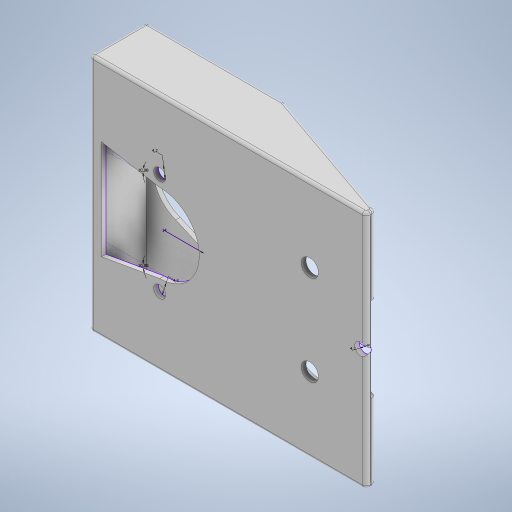
# Autodesk Inventor part: Tower
Saved by Autodesk Inventor 2024 (Build 280153000, 153)
## iProperties
Created: 2025-05-21
Part Number: Tower
Material: Ogólny
Document SubType Name: Modeling
Designer: Victoria
Density: 1 g/cm^3
Appearance: Domyślna
Author: Victoria
Autodesk Inventor part; units mm, degrees
ref_plane "YZ Plane" through (0, 0, 0) normal (1, 0, 0) x (0, 1, 0)
ref_plane "XZ Plane" through (0, 0, 0) normal (0, 1, 0) x (-1, 0, 0)
ref_plane "XY Plane" through (0, 0, 0) normal (0, 0, 1) x (1, 0, 0)
sketch "Szkic1" plane through (0, 0, 0) normal (0, 0, 1) x (1, 0, 0)
  circle A0 centre (0, 16) radius 3
  circle A1 centre (0, -16) radius 3
  line L0 (0, 0) -> (20, 0)
  line L1 (20, 0) -> (20, -42.5)
  line L2 (20, 0) -> (20, 42.5)
  line L3 (20, 0) -> (62.5, 0) construction
  line L4 (20, 42.5) -> (-78, 42.5)
  line L5 (-78, 42.5) -> (-78, -42.5)
  line L6 (-78, -42.5) -> (20, -42.5)
  dimension "d0" = 6
  dimension "d1" = 6
  dimension "d5" = 20
  dimension "d6" = 42.5
  dimension "d7" = 42.5
  dimension "d8" = 90
  dimension "d9" = 98
  dimension "d10" = 85
  dimension "d11" = 90
  constraints: 14 end point, 4 perpendicular, 2 centre point, 2 horizontal, 1 vertical
  measures "d0" diameter of A0
  measures "d1" diameter of A1
  measures "d5" distance of L0.start L0.end
  measures "d6" distance of L0.end L1.end
  measures "d7" distance of L0.end L2.end
  measures "d8" angle of L3 L2
  measures "d9" distance of L2.end L4.end
  measures "d10" distance of L4.end L5.end
  measures "d11" angle of L5 L4
extrude "Wyciągnięcie proste1" add sketch "Szkic1" along normal blind 1.6
sketch "Szkic6" plane through (0, 0, 0) normal (0, 0, -1) x (-1, 0, 0)
  line L0 (-18, 0) -> (53.3, 0)
  circle A0 centre (53.3, -18) radius 2.1
  circle A1 centre (53.3, 18) radius 2.1
  arc A2 (53.3, 14) -> (53.3, -14) centre (53.3, 0) ccw
  line L1 (53.3, -14) -> (74, -17.65)
  line L2 (78, 42.5) -> (78, -42.5) projected
  line L3 (53.3, -14) -> (78.381, -14) construction
  line L4 (53.3, 14) -> (74, 17.65)
  line L5 (53.3, 14) -> (78.381, 14) construction
  line L6 (78, 18.3553) -> (78, -18.3553)
  line L7 (74, -17.65) -> (74, 17.65)
  line L8 (78, 18.3553) -> (78, -18.3553)
  circle A3 centre (-18, 0) radius 2.1
  point P0 (0, 0)
  point P1 (78, 40.5)
  point P2 (78, -40.5)
  point P3 (74, 17.65)
  dimension "d50" = 4.2
  dimension "d52" = 4.2
  dimension "d53" = 14
  dimension "d54" = 10
  dimension "d55" = 10
  dimension "d103" = 4.2
  constraints: 16 end point, 4 centre point, 3 horizontal, 2 coincident, 2 point on circle, 2 point on line, 1 collinear, 1 parallel
  measures "d50" diameter of A0
  measures "d52" diameter of A1
  measures "d53" radius of A2
  measures "d54" angle of L1 L3
  measures "d55" angle of L5 L4
  measures "d103" diameter of A3
extrude "Wyciągnięcie proste6" cut sketch "Szkic6" against normal blind 8
sketch "Szkic15" plane through (0, 0, 0) normal (0, 0, -1) x (-1, 0, 0)
  line L0 (78, -42.5) -> (-20, -42.5) projected
  line L1 (78, -42.5) -> (78, 42.5)
  line L2 (78, 42.5) -> (-20, 42.5)
  line L3 (-20, 42.5) -> (-20, 41)
  line L4 (-20, 41) -> (76.5, 41)
  line L5 (76.5, 41) -> (76.5, -41)
  line L6 (76.5, -41) -> (-20, -41)
  line L7 (-20, -41) -> (-20, -42.5)
  line L8 (-20, -41) -> (-20, -42.5)
  line L9 (-20, -42.5) -> (78, -42.5)
  point P0 (0, 0)
  dimension "d104" = 1.5
  dimension "d105" = 96.5
  dimension "d106" = 82
  constraints: 18 end point, 5 perpendicular, 2 point on line, 1 collinear, 1 parallel
  measures "d104" distance of L2.end L3.end
  measures "d105" distance of L3.end L4.end
  measures "d106" distance of L4.end L5.end
extrude "Wyciągnięcie proste15" add sketch "Szkic15" along normal blind 16.8
sketch "Szkic16" plane through (0, 0, -16.8) normal (0, 0, -1) x (-1, 0, 0)
  line L0 (78, 42.5) -> (-20, 42.5) projected
  line L1 (-20, -42.5) -> (78, -42.5) projected
  line L2 (78, 42.5) -> (-20, 42.5)
  line L3 (-20, 42.5) -> (-20, -42.5)
  line L4 (-20, -42.5) -> (78, -42.5)
  line L5 (78, -42.5) -> (78, 42.5)
  point P0 (0, 0)
  constraints: 8 end point, 2 parallel, 1 horizontal, 1 perpendicular
extrude "Wyciągnięcie proste16" add sketch "Szkic16" along normal blind 1.6
sketch "Szkic17" plane through (-78, 42.5, 1.6) normal (0, 1, 0) x (1, 0, 0)
  line L0 (0, 0) -> (98, 0) projected
  line L1 (98, 0) -> (98, 3)
  line L2 (98, 0) -> (98, 20) projected
  line L3 (49, 20) -> (98, 3)
  line L4 (98, 20) -> (0, 20) projected
  line L5 (49, 20) -> (98, 20)
  line L6 (98, 20) -> (98, 3)
  point P0 (78, 1.6)
  dimension "d111" = 3
  constraints: 8 end point, 1 collinear, 1 point on line
  measures "d111" distance of L0.end L1.end
extrude "Wyciągnięcie proste17" cut sketch "Szkic17" against normal through all
sketch "Szkic18" plane through (-78, 42.5, 1.6) normal (0, 1, 0) x (1, 0, 0)
  line L0 (49, 20) -> (0, 20) projected
  line L1 (49, 20) -> (49, 18.6)
  line L2 (1.5, 1.6) -> (98, 1.6) projected
  line L3 (98, 1.6) -> (49, 18.6)
  line L4 (49, 18.6) -> (45.4326, 20)
  line L5 (45.4326, 20) -> (49, 20)
  line L6 (98, 3) -> (49, 20) projected
  line L7 (49, 20) -> (98, 3)
  line L8 (98, 3) -> (98, 1.6)
  point P0 (78, 1.6)
  dimension "d114" = 1.4
  constraints: 12 end point, 2 collinear, 1 perpendicular, 1 point on line, 1 vertical
  measures "d114" distance of L0.start L1.end
extrude "Wyciągnięcie proste18" add sketch "Szkic18" against normal up to surface (85 mm away)
sketch "Szkic19" plane through (0, 0, -18.4) normal (0, 0, -1) x (-1, 0, 0)
  line L0 (-20, -42.5) -> (-20, 42.5) projected
  line L1 (-20, 15) -> (-8, 15)
  line L2 (-8, 15) -> (-8, -15)
  line L3 (-8, -15) -> (-20, -15)
  line L4 (-20, -15) -> (-20, 15)
  point P0 (0, 0)
  dimension "d121" = 12
  dimension "d122" = 30
  constraints: 8 end point, 2 parallel, 1 horizontal, 1 perpendicular, 1 point on line
  measures "d121" distance of L2.end L3.end
  measures "d122" distance of L1.end L2.end
extrude "Wyciągnięcie proste19" cut sketch "Szkic19" against normal blind 18.4
sketch "Szkic20" plane through (0, 0, -18.4) normal (0, 0, -1) x (-1, 0, 0)
  circle A0 centre (0, 16) radius 3 projected
  circle A1 centre (0, -16) radius 3 projected
  arc A2 (-20, -0.6403) -> (-20, 0.6403) centre (-18, 0) ccw projected
  line L0 (-20, 0.6403) -> (-20, 42.5) projected
  line L1 (-20, 42.5) -> (78, 42.5) projected
  line L2 (78, 42.5) -> (78, -42.5) projected
  line L3 (78, -42.5) -> (-20, -42.5) projected
  line L4 (-20, -42.5) -> (-20, -0.6403) projected
  line L5 (74, 17.65) -> (53.3, 14) projected
  arc A3 (53.3, 14) -> (53.3, -14) centre (53.3, 0) ccw projected
  line L6 (53.3, -14) -> (74, -17.65) projected
  line L7 (74, -17.65) -> (74, 17.65) projected
  circle A4 centre (53.3, 18) radius 2.1 projected
  circle A5 centre (53.3, -18) radius 2.1 projected
  line L8 (74, 17.65) -> (74, -17.65) projected
  line L9 (29.8442, 27.4715) -> (51.0056, 18.1609)
  arc A6 (54.9687, 16.4172) -> (51.0056, 18.1609) centre (53.3, 18) ccw
  line L10 (54.9687, 16.4172) -> (66.0389, 11.5465)
  arc A7 (66.0389, -11.5465) -> (66.0389, 11.5465) centre (61.8, 0) ccw
  line L11 (66.0389, -11.5465) -> (54.9687, -16.4172)
  arc A8 (51.0056, -18.1609) -> (54.9687, -16.4172) centre (53.3, -18) ccw
  line L12 (51.0056, -18.1609) -> (29.8442, -27.4715)
  arc A9 (29.8442, 27.4715) -> (29.8442, -27.4715) centre (17.3, 0) ccw
  point P0 (0, 0)
  point P1 (74, -1.5652)
  point P2 (74, 1.5652)
  constraints: 8 end point, 8 point on circle, 4 centre point, 2 coincident
extrude "Wyciągnięcie proste20" cut sketch "Szkic20" against normal up to surface (18.4 mm away) contours A0 | A1 | L10 A7 L7 L11 L6 A3 L5 | L5 A3 L6 L11 A8 L12 A9 L9 A6 L10 | A4 | A5
fillet "Zaokrąglenie7" radius 1.4 6 edges at (20, 41.75, -1.4) (20, 28, -1.4) (20, 21.5702, 1.6) (20, -28, -1.4) (20, -41.75, -1.4) (20, -21.5702, 1.6)
fillet "Zaokrąglenie8" radius 1 18 edges at (19.5899, 42.5, 1.1899) (20, 42.5, -0.2019) (20, 42.5, 0.1) (19.7407, 42.5, -1.2155) (-4.9706, 42.5, -10.0633) (-29.7, 42.5, 1.6) (19.7407, -42.5, -1.2155) (20, -42.5, -0.2019) (20, -42.5, 0.1) (19.5899, -42.5, 1.1899) (-29.7, -42.5, 1.6) (-4.9706, -42.5, -10.0633) (-53.5, -42.5, -18.4) (-53.5, 42.5, -18.4) (-78, 42.5, -8.4) (-78, 0, 1.6) (-78, 0, -18.4) (-78, -42.5, -8.4)
sketch "Szkic21" plane through (19.0589, 15, -1.7265) normal (0.3277727, 0, -0.9447566) x (-0.9447566, 0, -0.3277727)
  line L0 (0, 26.5) -> (50.8691, 26.5) projected
  line L1 (0, 0) -> (0, 26.5) projected
  line L2 (50.8691, 26.5) -> (0, 26.5)
  line L3 (0, 26.5) -> (0, 0)
  line L4 (0, 0) -> (50.8691, 0)
  line L5 (50.8691, 0) -> (50.8691, 26.5)
  line L6 (0, -56.5) -> (50.8691, -56.5)
  line L7 (50.8691, -56.5) -> (50.8691, -30)
  line L8 (50.8691, -30) -> (0, -30)
  line L9 (0, -30) -> (0, -56.5)
  line L10 (47.8691, 3) -> (3, 3)
  line L11 (3, 3) -> (3, 23.5)
  line L12 (3, 23.5) -> (47.8691, 23.5)
  line L13 (47.8691, 23.5) -> (47.8691, 3)
  line L14 (47.8691, -33) -> (47.8691, -53.5)
  line L15 (47.8691, -53.5) -> (3, -53.5)
  line L16 (3, -53.5) -> (3, -33)
  line L17 (3, -33) -> (47.8691, -33)
  line L18 (50.8691, 13.25) -> (98.7381, 13.25) construction
  line L19 (4.5, 22) -> (7.5, 22)
  line L20 (7.5, 22) -> (7.5, 4.5)
  line L21 (7.5, 4.5) -> (4.5, 4.5)
  line L22 (4.5, 4.5) -> (4.5, 22)
  line L23 (4.5, 22) -> (7.5, 4.5) construction
  line L24 (7.5, 22) -> (4.5, 4.5) construction
  line L25 (13, 22) -> (10, 22)
  line L26 (10, 22) -> (10, 4.5)
  line L27 (10, 4.5) -> (13, 4.5)
  line L28 (13, 4.5) -> (13, 22)
  line L29 (13, 22) -> (10, 4.5) construction
  line L30 (10, 22) -> (13, 4.5) construction
  line L31 (14.5, 22) -> (14.5, 4.5)
  line L32 (17.5, 22) -> (14.5, 22)
  line L33 (17.5, 4.5) -> (17.5, 22)
  line L34 (14.5, 4.5) -> (17.5, 4.5)
  line L35 (19, 22) -> (19, 4.5)
  line L36 (22, 22) -> (19, 22)
  line L37 (22, 4.5) -> (22, 22)
  line L38 (19, 4.5) -> (22, 4.5)
  line L39 (7.5, -34.5) -> (4.5, -34.5)
  line L40 (4.5, -34.5) -> (4.5, -52)
  line L41 (4.5, -52) -> (7.5, -52)
  line L42 (7.5, -52) -> (7.5, -34.5)
  line L43 (7.5, -34.5) -> (4.5, -52) construction
  line L44 (4.5, -34.5) -> (7.5, -52) construction
  line L45 (13, -34.5) -> (10, -34.5)
  line L46 (10, -34.5) -> (10, -52)
  line L47 (10, -52) -> (13, -52)
  line L48 (13, -52) -> (13, -34.5)
  line L49 (13, -34.5) -> (10, -52) construction
  line L50 (10, -34.5) -> (13, -52) construction
  point P0 (17.4401, -15)
  point P1 (6, 13.25)
  point P2 (11.5, 13.25)
  point P3 (6, -43.25)
  point P4 (11.5, -43.25)
  dimension "d133" = 26.5
  dimension "d134" = 26.5
  dimension "d135" = 3
  dimension "d136" = 3
  dimension "d138" = 3
  dimension "d139" = 3
  dimension "d140" = 17.5
  dimension "d141" = 17.5
  dimension "d148" = 4.5
  dimension "d154" = 17.5
  dimension "d155" = 3
  constraints: 98 end point, 16 parallel, 9 midpoint, 8 horizontal, 8 perpendicular, 3 point on line, 22 other
  measures "d133" distance of L4.end L0.end
  measures "d134" distance of L6.end L7.end
  measures "d135" distance between parallel lines of L4 L10
  measures "d136" distance between parallel lines of L7 L14
  measures "d138" distance of L20.end L21.end
  measures "d139" distance of L27.end L26.end
  measures "d140" distance of L26.end L25.end
  measures "d141" distance of L21.end L19.start
  measures "d148" distance of L25.end L31.start
  measures "d154" distance of L40.end L39.end
  measures "d155" distance of L47.end L46.end
extrude "Wyciągnięcie proste21" cut sketch "Szkic21" against normal blind 0.5 contours L10 L11 L12 L13 | L14 L15 L16 L17 | L32 L33 L34 L31 | L36 L37 L38 L35
